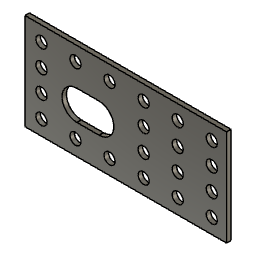
plate_3 v2 (Autodesk Fusion 360 design; units mm, degrees)
Autodesk Fusion 360 part; units mm, degrees
sketch "Sketch1" plane through (0, 0, 0) normal (0, 1, 0) x (1, 0, 0)
  line L0 (0, 0) -> (272.2, 0)
  line L1 (272.2, 0) -> (272.2, -130)
  line L2 (272.2, -130) -> (0, -130)
  line L3 (0, -130) -> (0, 0)
  dimension "d1" = 272.2
  dimension "d2" = 130
  constraint horizontal L0
  constraint vertical L1
  constraint horizontal L2
  constraint vertical L3
  constraint coincident L0.start L3.end
  measures "d1" distance of L0.start L0.end
  measures "d2" distance of L0.start L2.end
extrude "Extrude1" add sketch "Sketch1" against normal blind 6
sketch "Sketch2" plane through (0, -6, 0) normal (0, -1, 0) x (1, 0, 0)
  line L0 (272.2, 130) -> (0, 130)
  line L1 (0, 130) -> (0, 0)
  line L2 (0, 0) -> (272.2, 0)
  line L3 (272.2, 0) -> (272.2, 130)
  line L4 (70, 40) -> (100, 40)
  arc A0 (100, 40) -> (100, 80) centre (100, 60) ccw
  line L5 (100, 80) -> (70, 80)
  arc A1 (70, 80) -> (70, 40) centre (70, 60) ccw
  line L6 (50, 60) -> (120, 60) construction
  circle A2 centre (252.2, 110) radius 7.5
  circle A3 centre (206.2, 110) radius 7.5
  circle A4 centre (160.2, 110) radius 7.5
  circle A5 centre (114.2, 110) radius 7.5
  circle A6 centre (68.2, 110) radius 7.5
  circle A7 centre (252.2, 80) radius 7.5
  circle A8 centre (206.2, 80) radius 7.5
  circle A9 centre (252.2, 50) radius 7.5
  circle A10 centre (206.2, 50) radius 7.5
  circle A11 centre (160.2, 50) radius 7.5
  circle A12 centre (22.2, 110) radius 7.5
  circle A13 centre (22.2, 80) radius 7.5
  circle A14 centre (22.2, 50) radius 7.5
  circle A15 centre (252.2, 20) radius 7.5
  circle A16 centre (206.2, 20) radius 7.5
  circle A17 centre (160.2, 20) radius 7.5
  circle A18 centre (114.2, 20) radius 7.5
  circle A19 centre (68.2, 20) radius 7.5
  circle A20 centre (22.2, 20) radius 7.5
  circle A21 centre (160.2, 80) radius 7.5
  dimension "d5" = 40
  dimension "d6" = 50
  dimension "d8" = 40
  dimension "d9" = 15
  dimension "d10" = 20
  dimension "d11" = 20
  dimension "d14" = -230
  dimension "d15" = -90
  constraint tangent L4 A0
  constraint tangent A0 L5
  constraint parallel L4 L5
  constraint tangent L4 A1
  constraint midpoint A1 L6.start
  constraint midpoint A0 L6.end
  measures "d5" diameter of A0
  measures "d6" distance of L1 L6.start
  measures "d8" distance of L2 L4
  measures "d9" diameter of A2
  measures "d10" distance of L0 A2.centre
  measures "d11" distance of L3 A2.centre
extrude "Extrude2" cut sketch "Sketch2" against normal up to surface (6 mm away) contours L4 A0 L5 A1 | A2 | A3 | A4 | A5 | A6 | A7 | A8 | A9 | A10 | A11 | A12 | A13 | A14 | A15 | A16 | A17 | A18 | A19 | A20 | A21
